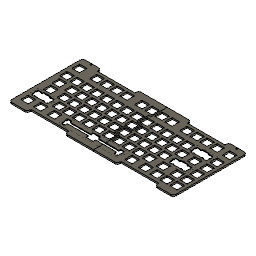
Plate (Autodesk Fusion 360 design; units mm, degrees)
part number: 2026-05-10-17-46-24-524
Autodesk Fusion 360 part; units mm, degrees
(part 1 of 4)
sketch "Plate May 11 2026" plane through (0, 0, 0) normal (0, 0, 1) x (1, 0, 0)
  line L0 (3.025, -2.525) -> (16.025, -2.525)
  line L1 (3.025, -16.525) -> (16.025, -16.525)
  line L2 (2.525, -3.025) -> (2.525, -16.025)
  line L3 (16.525, -3.025) -> (16.525, -16.025)
  arc A0 (3.025, -2.525) -> (2.525, -3.025) centre (3.025, -3.025) ccw
  arc A1 (16.525, -3.025) -> (16.025, -2.525) centre (16.025, -3.025) ccw
  arc A2 (2.525, -16.025) -> (3.025, -16.525) centre (3.025, -16.025) ccw
  arc A3 (16.025, -16.525) -> (16.525, -16.025) centre (16.025, -16.025) ccw
  line L4 (36.3625, -2.525) -> (49.3625, -2.525)
  line L5 (36.3625, -16.525) -> (49.3625, -16.525)
  line L6 (35.8625, -3.025) -> (35.8625, -16.025)
  line L7 (49.8625, -3.025) -> (49.8625, -16.025)
  arc A4 (36.3625, -2.525) -> (35.8625, -3.025) centre (36.3625, -3.025) ccw
  arc A5 (49.8625, -3.025) -> (49.3625, -2.525) centre (49.3625, -3.025) ccw
  arc A6 (35.8625, -16.025) -> (36.3625, -16.525) centre (36.3625, -16.025) ccw
  arc A7 (49.3625, -16.525) -> (49.8625, -16.025) centre (49.3625, -16.025) ccw
  line L8 (55.4125, -2.525) -> (68.4125, -2.525)
  line L9 (55.4125, -16.525) -> (68.4125, -16.525)
  line L10 (54.9125, -3.025) -> (54.9125, -16.025)
  line L11 (68.9125, -3.025) -> (68.9125, -16.025)
  arc A8 (55.4125, -2.525) -> (54.9125, -3.025) centre (55.4125, -3.025) ccw
  arc A9 (68.9125, -3.025) -> (68.4125, -2.525) centre (68.4125, -3.025) ccw
  arc A10 (54.9125, -16.025) -> (55.4125, -16.525) centre (55.4125, -16.025) ccw
  arc A11 (68.4125, -16.525) -> (68.9125, -16.025) centre (68.4125, -16.025) ccw
  line L12 (74.4625, -2.525) -> (87.4625, -2.525)
  line L13 (74.4625, -16.525) -> (87.4625, -16.525)
  line L14 (73.9625, -3.025) -> (73.9625, -16.025)
  line L15 (87.9625, -3.025) -> (87.9625, -16.025)
  arc A12 (74.4625, -2.525) -> (73.9625, -3.025) centre (74.4625, -3.025) ccw
  arc A13 (87.9625, -3.025) -> (87.4625, -2.525) centre (87.4625, -3.025) ccw
  arc A14 (73.9625, -16.025) -> (74.4625, -16.525) centre (74.4625, -16.025) ccw
  arc A15 (87.4625, -16.525) -> (87.9625, -16.025) centre (87.4625, -16.025) ccw
  line L16 (93.5125, -2.525) -> (106.5125, -2.525)
  line L17 (93.5125, -16.525) -> (106.5125, -16.525)
  line L18 (93.0125, -3.025) -> (93.0125, -16.025)
  line L19 (107.0125, -3.025) -> (107.0125, -16.025)
  arc A16 (93.5125, -2.525) -> (93.0125, -3.025) centre (93.5125, -3.025) ccw
  arc A17 (107.0125, -3.025) -> (106.5125, -2.525) centre (106.5125, -3.025) ccw
  arc A18 (93.0125, -16.025) -> (93.5125, -16.525) centre (93.5125, -16.025) ccw
  arc A19 (106.5125, -16.525) -> (107.0125, -16.025) centre (106.5125, -16.025) ccw
  line L20 (122.0875, -2.525) -> (135.0875, -2.525)
  line L21 (122.0875, -16.525) -> (135.0875, -16.525)
  line L22 (121.5875, -3.025) -> (121.5875, -16.025)
  line L23 (135.5875, -3.025) -> (135.5875, -16.025)
  arc A20 (122.0875, -2.525) -> (121.5875, -3.025) centre (122.0875, -3.025) ccw
  arc A21 (135.5875, -3.025) -> (135.0875, -2.525) centre (135.0875, -3.025) ccw
  arc A22 (121.5875, -16.025) -> (122.0875, -16.525) centre (122.0875, -16.025) ccw
  arc A23 (135.0875, -16.525) -> (135.5875, -16.025) centre (135.0875, -16.025) ccw
  line L24 (141.1375, -2.525) -> (154.1375, -2.525)
  line L25 (141.1375, -16.525) -> (154.1375, -16.525)
  line L26 (140.6375, -3.025) -> (140.6375, -16.025)
  line L27 (154.6375, -3.025) -> (154.6375, -16.025)
  arc A24 (141.1375, -2.525) -> (140.6375, -3.025) centre (141.1375, -3.025) ccw
  arc A25 (154.6375, -3.025) -> (154.1375, -2.525) centre (154.1375, -3.025) ccw
  arc A26 (140.6375, -16.025) -> (141.1375, -16.525) centre (141.1375, -16.025) ccw
  arc A27 (154.1375, -16.525) -> (154.6375, -16.025) centre (154.1375, -16.025) ccw
  line L28 (160.1875, -2.525) -> (173.1875, -2.525)
  line L29 (160.1875, -16.525) -> (173.1875, -16.525)
  line L30 (159.6875, -3.025) -> (159.6875, -16.025)
  line L31 (173.6875, -3.025) -> (173.6875, -16.025)
  arc A28 (160.1875, -2.525) -> (159.6875, -3.025) centre (160.1875, -3.025) ccw
  arc A29 (173.6875, -3.025) -> (173.1875, -2.525) centre (173.1875, -3.025) ccw
  arc A30 (159.6875, -16.025) -> (160.1875, -16.525) centre (160.1875, -16.025) ccw
  arc A31 (173.1875, -16.525) -> (173.6875, -16.025) centre (173.1875, -16.025) ccw
  line L32 (179.2375, -2.525) -> (192.2375, -2.525)
  line L33 (179.2375, -16.525) -> (192.2375, -16.525)
  line L34 (178.7375, -3.025) -> (178.7375, -16.025)
  line L35 (192.7375, -3.025) -> (192.7375, -16.025)
  arc A32 (179.2375, -2.525) -> (178.7375, -3.025) centre (179.2375, -3.025) ccw
  arc A33 (192.7375, -3.025) -> (192.2375, -2.525) centre (192.2375, -3.025) ccw
  arc A34 (178.7375, -16.025) -> (179.2375, -16.525) centre (179.2375, -16.025) ccw
  arc A35 (192.2375, -16.525) -> (192.7375, -16.025) centre (192.2375, -16.025) ccw
  line L36 (207.8125, -2.525) -> (220.8125, -2.525)
  line L37 (207.8125, -16.525) -> (220.8125, -16.525)
  line L38 (207.3125, -3.025) -> (207.3125, -16.025)
  line L39 (221.3125, -3.025) -> (221.3125, -16.025)
  arc A36 (207.8125, -2.525) -> (207.3125, -3.025) centre (207.8125, -3.025) ccw
  arc A37 (221.3125, -3.025) -> (220.8125, -2.525) centre (220.8125, -3.025) ccw
  arc A38 (207.3125, -16.025) -> (207.8125, -16.525) centre (207.8125, -16.025) ccw
  arc A39 (220.8125, -16.525) -> (221.3125, -16.025) centre (220.8125, -16.025) ccw
  line L40 (226.8625, -2.525) -> (239.8625, -2.525)
  line L41 (226.8625, -16.525) -> (239.8625, -16.525)
  line L42 (226.3625, -3.025) -> (226.3625, -16.025)
  line L43 (240.3625, -3.025) -> (240.3625, -16.025)
  arc A40 (226.8625, -2.525) -> (226.3625, -3.025) centre (226.8625, -3.025) ccw
  arc A41 (240.3625, -3.025) -> (239.8625, -2.525) centre (239.8625, -3.025) ccw
  arc A42 (226.3625, -16.025) -> (226.8625, -16.525) centre (226.8625, -16.025) ccw
  arc A43 (239.8625, -16.525) -> (240.3625, -16.025) centre (239.8625, -16.025) ccw
  line L44 (245.9125, -2.525) -> (258.9125, -2.525)
  line L45 (245.9125, -16.525) -> (258.9125, -16.525)
  line L46 (245.4125, -3.025) -> (245.4125, -16.025)
  line L47 (259.4125, -3.025) -> (259.4125, -16.025)
  arc A44 (245.9125, -2.525) -> (245.4125, -3.025) centre (245.9125, -3.025) ccw
  arc A45 (259.4125, -3.025) -> (258.9125, -2.525) centre (258.9125, -3.025) ccw
  arc A46 (245.4125, -16.025) -> (245.9125, -16.525) centre (245.9125, -16.025) ccw
  arc A47 (258.9125, -16.525) -> (259.4125, -16.025) centre (258.9125, -16.025) ccw
  line L48 (264.9625, -2.525) -> (277.9625, -2.525)
  line L49 (264.9625, -16.525) -> (277.9625, -16.525)
  line L50 (264.4625, -3.025) -> (264.4625, -16.025)
  line L51 (278.4625, -3.025) -> (278.4625, -16.025)
  arc A48 (264.9625, -2.525) -> (264.4625, -3.025) centre (264.9625, -3.025) ccw
  arc A49 (278.4625, -3.025) -> (277.9625, -2.525) centre (277.9625, -3.025) ccw
  arc A50 (264.4625, -16.025) -> (264.9625, -16.525) centre (264.9625, -16.025) ccw
  arc A51 (277.9625, -16.525) -> (278.4625, -16.025) centre (277.9625, -16.025) ccw
  line L52 (288.775, -2.5211) -> (301.775, -2.521)
  line L53 (288.775, -16.5282) -> (301.775, -16.5283)
  line L54 (288.239, -3.025) -> (288.2473, -16.025)
  line L55 (302.2755, -3.025) -> (302.2758, -16.025)
  arc A52 (288.775, -2.5211) -> (288.239, -3.025) centre (288.7579, -3.04) ccw
  arc A53 (302.2755, -3.025) -> (301.775, -2.521) centre (301.7743, -3.0222) ccw
  arc A54 (288.2473, -16.025) -> (288.775, -16.5282) centre (288.7619, -16.0136) ccw
  arc A55 (301.775, -16.5283) -> (302.2758, -16.025) centre (301.7745, -16.0271) ccw
  line L56 (3.025, -26.3375) -> (16.025, -26.3375)
  line L57 (3.025, -40.3375) -> (16.025, -40.3375)
  line L58 (2.525, -26.8375) -> (2.525, -39.8375)
  line L59 (16.525, -26.8375) -> (16.525, -39.8375)
  arc A56 (3.025, -26.3375) -> (2.525, -26.8375) centre (3.025, -26.8375) ccw
  arc A57 (16.525, -26.8375) -> (16.025, -26.3375) centre (16.025, -26.8375) ccw
  arc A58 (2.525, -39.8375) -> (3.025, -40.3375) centre (3.025, -39.8375) ccw
  arc A59 (16.025, -40.3375) -> (16.525, -39.8375) centre (16.025, -39.8375) ccw
  line L60 (22.075, -26.3375) -> (35.075, -26.3375)
  line L61 (22.075, -40.3375) -> (35.075, -40.3375)
  line L62 (21.575, -26.8375) -> (21.575, -39.8375)
  line L63 (35.575, -26.8375) -> (35.575, -39.8375)
  arc A60 (22.075, -26.3375) -> (21.575, -26.8375) centre (22.075, -26.8375) ccw
  arc A61 (35.575, -26.8375) -> (35.075, -26.3375) centre (35.075, -26.8375) ccw
  arc A62 (21.575, -39.8375) -> (22.075, -40.3375) centre (22.075, -39.8375) ccw
  arc A63 (35.075, -40.3375) -> (35.575, -39.8375) centre (35.075, -39.8375) ccw
  line L64 (41.125, -26.3375) -> (54.125, -26.3375)
  line L65 (41.125, -40.3375) -> (54.125, -40.3375)
  line L66 (40.625, -26.8375) -> (40.625, -39.8375)
  line L67 (54.625, -26.8375) -> (54.625, -39.8375)
  arc A64 (41.125, -26.3375) -> (40.625, -26.8375) centre (41.125, -26.8375) ccw
  arc A65 (54.625, -26.8375) -> (54.125, -26.3375) centre (54.125, -26.8375) ccw
  arc A66 (40.625, -39.8375) -> (41.125, -40.3375) centre (41.125, -39.8375) ccw
  arc A67 (54.125, -40.3375) -> (54.625, -39.8375) centre (54.125, -39.8375) ccw
  line L68 (60.175, -26.3375) -> (73.175, -26.3375)
  line L69 (60.175, -40.3375) -> (73.175, -40.3375)
  line L70 (59.675, -26.8375) -> (59.675, -39.8375)
  line L71 (73.675, -26.8375) -> (73.675, -39.8375)
  arc A68 (60.175, -26.3375) -> (59.675, -26.8375) centre (60.175, -26.8375) ccw
  arc A69 (73.675, -26.8375) -> (73.175, -26.3375) centre (73.175, -26.8375) ccw
  arc A70 (59.675, -39.8375) -> (60.175, -40.3375) centre (60.175, -39.8375) ccw
  arc A71 (73.175, -40.3375) -> (73.675, -39.8375) centre (73.175, -39.8375) ccw
  line L72 (79.225, -26.3375) -> (92.225, -26.3375)
  line L73 (79.225, -40.3375) -> (92.225, -40.3375)
  line L74 (78.725, -26.8375) -> (78.725, -39.8375)
  line L75 (92.725, -26.8375) -> (92.725, -39.8375)
  arc A72 (79.225, -26.3375) -> (78.725, -26.8375) centre (79.225, -26.8375) ccw
  arc A73 (92.725, -26.8375) -> (92.225, -26.3375) centre (92.225, -26.8375) ccw
  arc A74 (78.725, -39.8375) -> (79.225, -40.3375) centre (79.225, -39.8375) ccw
  arc A75 (92.225, -40.3375) -> (92.725, -39.8375) centre (92.225, -39.8375) ccw
  line L76 (98.275, -26.3375) -> (111.275, -26.3375)
  line L77 (98.275, -40.3375) -> (111.275, -40.3375)
  line L78 (97.775, -26.8375) -> (97.775, -39.8375)
  line L79 (111.775, -26.8375) -> (111.775, -39.8375)
  arc A76 (98.275, -26.3375) -> (97.775, -26.8375) centre (98.275, -26.8375) ccw
  arc A77 (111.775, -26.8375) -> (111.275, -26.3375) centre (111.275, -26.8375) ccw
  arc A78 (97.775, -39.8375) -> (98.275, -40.3375) centre (98.275, -39.8375) ccw
  arc A79 (111.275, -40.3375) -> (111.775, -39.8375) centre (111.275, -39.8375) ccw
  line L80 (117.325, -26.3375) -> (130.325, -26.3375)
  line L81 (117.325, -40.3375) -> (130.325, -40.3375)
  line L82 (116.825, -26.8375) -> (116.825, -39.8375)
  line L83 (130.825, -26.8375) -> (130.825, -39.8375)
  arc A80 (117.325, -26.3375) -> (116.825, -26.8375) centre (117.325, -26.8375) ccw
  arc A81 (130.825, -26.8375) -> (130.325, -26.3375) centre (130.325, -26.8375) ccw
  arc A82 (116.825, -39.8375) -> (117.325, -40.3375) centre (117.325, -39.8375) ccw
  arc A83 (130.325, -40.3375) -> (130.825, -39.8375) centre (130.325, -39.8375) ccw
  line L84 (136.375, -26.3375) -> (149.375, -26.3375)
  line L85 (136.375, -40.3375) -> (149.375, -40.3375)
  line L86 (135.875, -26.8375) -> (135.875, -39.8375)
  line L87 (149.875, -26.8375) -> (149.875, -39.8375)
  arc A84 (136.375, -26.3375) -> (135.875, -26.8375) centre (136.375, -26.8375) ccw
  arc A85 (149.875, -26.8375) -> (149.375, -26.3375) centre (149.375, -26.8375) ccw
  arc A86 (135.875, -39.8375) -> (136.375, -40.3375) centre (136.375, -39.8375) ccw
  arc A87 (149.375, -40.3375) -> (149.875, -39.8375) centre (149.375, -39.8375) ccw
  line L88 (155.425, -26.3375) -> (168.425, -26.3375)
  line L89 (155.425, -40.3375) -> (168.425, -40.3375)
  line L90 (154.925, -26.8375) -> (154.925, -39.8375)
  line L91 (168.925, -26.8375) -> (168.925, -39.8375)
  arc A88 (155.425, -26.3375) -> (154.925, -26.8375) centre (155.425, -26.8375) ccw
  arc A89 (168.925, -26.8375) -> (168.425, -26.3375) centre (168.425, -26.8375) ccw
  arc A90 (154.925, -39.8375) -> (155.425, -40.3375) centre (155.425, -39.8375) ccw
  arc A91 (168.425, -40.3375) -> (168.925, -39.8375) centre (168.425, -39.8375) ccw
  line L92 (174.475, -26.3375) -> (187.475, -26.3375)
  line L93 (174.475, -40.3375) -> (187.475, -40.3375)
  line L94 (173.975, -26.8375) -> (173.975, -39.8375)
  line L95 (187.975, -26.8375) -> (187.975, -39.8375)
  arc A92 (174.475, -26.3375) -> (173.975, -26.8375) centre (174.475, -26.8375) ccw
  arc A93 (187.975, -26.8375) -> (187.475, -26.3375) centre (187.475, -26.8375) ccw
  arc A94 (173.975, -39.8375) -> (174.475, -40.3375) centre (174.475, -39.8375) ccw
  arc A95 (187.475, -40.3375) -> (187.975, -39.8375) centre (187.475, -39.8375) ccw
  line L96 (193.525, -26.3375) -> (206.525, -26.3375)
  line L97 (193.525, -40.3375) -> (206.525, -40.3375)
  line L98 (193.025, -26.8375) -> (193.025, -39.8375)
  line L99 (207.025, -26.8375) -> (207.025, -39.8375)
  arc A96 (193.525, -26.3375) -> (193.025, -26.8375) centre (193.525, -26.8375) ccw
  arc A97 (207.025, -26.8375) -> (206.525, -26.3375) centre (206.525, -26.8375) ccw
  arc A98 (193.025, -39.8375) -> (193.525, -40.3375) centre (193.525, -39.8375) ccw
  arc A99 (206.525, -40.3375) -> (207.025, -39.8375) centre (206.525, -39.8375) ccw
  line L100 (212.575, -26.3375) -> (225.575, -26.3375)
  line L101 (212.575, -40.3375) -> (225.575, -40.3375)
  line L102 (212.075, -26.8375) -> (212.075, -39.8375)
  line L103 (226.075, -26.8375) -> (226.075, -39.8375)
  arc A100 (212.575, -26.3375) -> (212.075, -26.8375) centre (212.575, -26.8375) ccw
  arc A101 (226.075, -26.8375) -> (225.575, -26.3375) centre (225.575, -26.8375) ccw
  arc A102 (212.075, -39.8375) -> (212.575, -40.3375) centre (212.575, -39.8375) ccw
  arc A103 (225.575, -40.3375) -> (226.075, -39.8375) centre (225.575, -39.8375) ccw
  line L104 (231.625, -26.3375) -> (244.625, -26.3375)
  line L105 (231.625, -40.3375) -> (244.625, -40.3375)
  line L106 (231.125, -26.8375) -> (231.125, -39.8375)
  line L107 (245.125, -26.8375) -> (245.125, -39.8375)
  arc A104 (231.625, -26.3375) -> (231.125, -26.8375) centre (231.625, -26.8375) ccw
  arc A105 (245.125, -26.8375) -> (244.625, -26.3375) centre (244.625, -26.8375) ccw
  arc A106 (231.125, -39.8375) -> (231.625, -40.3375) centre (231.625, -39.8375) ccw
  arc A107 (244.625, -40.3375) -> (245.125, -39.8375) centre (244.625, -39.8375) ccw
  line L108 (260.2, -26.3375) -> (273.2, -26.3375)
  line L109 (260.2, -40.3375) -> (273.2, -40.3375)
  line L110 (259.7, -26.8375) -> (259.7, -39.8375)
  line L111 (273.7, -26.8375) -> (273.7, -39.8375)
  arc A108 (260.2, -26.3375) -> (259.7, -26.8375) centre (260.2, -26.8375) ccw
  arc A109 (273.7, -26.8375) -> (273.2, -26.3375) centre (273.2, -26.8375) ccw
  arc A110 (259.7, -39.8375) -> (260.2, -40.3375) centre (260.2, -39.8375) ccw
  arc A111 (273.2, -40.3375) -> (273.7, -39.8375) centre (273.2, -39.8375) ccw
  line L112 (251.9346, -27.6479) -> (257.5894, -27.6479)
  line L113 (258.0894, -28.1479) -> (258.0894, -28.4607)
  line L114 (258.0894, -28.4607) -> (266.7, -28.4607)
  line L115 (266.7, -39.1541) -> (258.5894, -39.1541)
  line L116 (258.0894, -39.6541) -> (258.0894, -39.9415)
  line L117 (258.0894, -39.9415) -> (256.786, -39.9415)
  line L118 (256.286, -40.4415) -> (256.286, -40.6099)
  line L119 (255.786, -41.1099) -> (253.738, -41.1099)
  line L120 (253.238, -40.6099) -> (253.238, -40.4415)
  line L121 (252.738, -39.9415) -> (251.9346, -39.9415)
  line L122 (251.4346, -39.4415) -> (251.4346, -34.3455)
  line L123 (250.9346, -33.8455) -> (250.571, -33.8455)
  line L124 (250.571, -33.8455) -> (250.571, -31.5515)
  line L125 (251.071, -31.0515) -> (251.4346, -31.0515)
  line L126 (251.4346, -31.0515) -> (251.4346, -28.1479)
  arc A112 (258.0894, -28.1479) -> (257.5894, -27.6479) centre (257.5894, -28.1479) ccw
  arc A113 (258.5894, -39.1541) -> (258.0894, -39.6541) centre (258.5894, -39.6541) ccw
  arc A114 (256.786, -39.9415) -> (256.286, -40.4415) centre (256.786, -40.4415) ccw
  arc A115 (255.786, -41.1099) -> (256.286, -40.6099) centre (255.786, -40.6099) ccw
  arc A116 (253.238, -40.6099) -> (253.738, -41.1099) centre (253.738, -40.6099) ccw
  arc A117 (253.238, -40.4415) -> (252.738, -39.9415) centre (252.738, -40.4415) ccw
  arc A118 (251.4346, -39.4415) -> (251.9346, -39.9415) centre (251.9346, -39.4415) ccw
  arc A119 (251.4346, -34.3455) -> (250.9346, -33.8455) centre (250.9346, -34.3455) ccw
  arc A120 (251.071, -31.0515) -> (250.571, -31.5515) centre (251.071, -31.5515) ccw
  arc A121 (251.9346, -27.6479) -> (251.4346, -28.1479) centre (251.9346, -28.1479) ccw
  line L127 (281.4654, -27.6479) -> (275.8106, -27.6479)
  line L128 (275.3106, -28.1479) -> (275.3106, -28.4607)
  line L129 (275.3106, -28.4607) -> (266.7, -28.4607)
  line L130 (266.7, -39.1541) -> (274.8106, -39.1541)
  line L131 (275.3106, -39.6541) -> (275.3106, -39.9415)
  line L132 (275.3106, -39.9415) -> (276.614, -39.9415)
  line L133 (277.114, -40.4415) -> (277.114, -40.6099)
  line L134 (277.614, -41.1099) -> (279.662, -41.1099)
  line L135 (280.162, -40.6099) -> (280.162, -40.4415)
  line L136 (280.662, -39.9415) -> (281.4654, -39.9415)
  line L137 (281.9654, -39.4415) -> (281.9654, -34.3455)
  line L138 (282.4654, -33.8455) -> (282.829, -33.8455)
  line L139 (282.829, -33.8455) -> (282.829, -31.5515)
  line L140 (282.329, -31.0515) -> (281.9654, -31.0515)
  line L141 (281.9654, -31.0515) -> (281.9654, -28.1479)
  arc A122 (275.8106, -27.6479) -> (275.3106, -28.1479) centre (275.8106, -28.1479) ccw
  arc A123 (275.3106, -39.6541) -> (274.8106, -39.1541) centre (274.8106, -39.6541) ccw
  arc A124 (277.114, -40.4415) -> (276.614, -39.9415) centre (276.614, -40.4415) ccw
  arc A125 (277.114, -40.6099) -> (277.614, -41.1099) centre (277.614, -40.6099) ccw
  arc A126 (279.662, -41.1099) -> (280.162, -40.6099) centre (279.662, -40.6099) ccw
  arc A127 (280.662, -39.9415) -> (280.162, -40.4415) centre (280.662, -40.4415) ccw
  arc A128 (281.4654, -39.9415) -> (281.9654, -39.4415) centre (281.4654, -39.4415) ccw
  arc A129 (282.4654, -33.8455) -> (281.9654, -34.3455) centre (282.4654, -34.3455) ccw
  arc A130 (282.829, -31.5515) -> (282.329, -31.0515) centre (282.329, -31.5515) ccw
  arc A131 (281.9654, -28.1479) -> (281.4654, -27.6479) centre (281.4654, -28.1479) ccw
  line L142 (288.775, -26.3375) -> (301.775, -26.3375)
  line L143 (288.775, -40.3375) -> (301.775, -40.3375)
  line L144 (288.275, -26.8375) -> (288.275, -39.8375)
  line L145 (302.275, -26.8375) -> (302.275, -39.8375)
  arc A132 (288.775, -26.3375) -> (288.275, -26.8375) centre (288.775, -26.8375) ccw
  arc A133 (302.275, -26.8375) -> (301.775, -26.3375) centre (301.775, -26.8375) ccw
  arc A134 (288.275, -39.8375) -> (288.775, -40.3375) centre (288.775, -39.8375) ccw
  arc A135 (301.775, -40.3375) -> (302.275, -39.8375) centre (301.775, -39.8375) ccw
  line L146 (7.7875, -45.3875) -> (20.7875, -45.3875)
  line L147 (7.7875, -59.3875) -> (20.7875, -59.3875)
  line L148 (7.2875, -45.8875) -> (7.2875, -58.8875)
  line L149 (21.2875, -45.8875) -> (21.2875, -58.8875)
  arc A136 (7.7875, -45.3875) -> (7.2875, -45.8875) centre (7.7875, -45.8875) ccw
  arc A137 (21.2875, -45.8875) -> (20.7875, -45.3875) centre (20.7875, -45.8875) ccw
  arc A138 (7.2875, -58.8875) -> (7.7875, -59.3875) centre (7.7875, -58.8875) ccw
  arc A139 (20.7875, -59.3875) -> (21.2875, -58.8875) centre (20.7875, -58.8875) ccw
  line L150 (31.6, -45.3875) -> (44.6, -45.3875)
  line L151 (31.6, -59.3875) -> (44.6, -59.3875)
  line L152 (31.1, -45.8875) -> (31.1, -58.8875)
  line L153 (45.1, -45.8875) -> (45.1, -58.8875)
  arc A140 (31.6, -45.3875) -> (31.1, -45.8875) centre (31.6, -45.8875) ccw
  arc A141 (45.1, -45.8875) -> (44.6, -45.3875) centre (44.6, -45.8875) ccw
  arc A142 (31.1, -58.8875) -> (31.6, -59.3875) centre (31.6, -58.8875) ccw
  arc A143 (44.6, -59.3875) -> (45.1, -58.8875) centre (44.6, -58.8875) ccw
  line L154 (50.65, -45.3875) -> (63.65, -45.3875)
  line L155 (50.65, -59.3875) -> (63.65, -59.3875)
  line L156 (50.15, -45.8875) -> (50.15, -58.8875)
  line L157 (64.15, -45.8875) -> (64.15, -58.8875)
  arc A144 (50.65, -45.3875) -> (50.15, -45.8875) centre (50.65, -45.8875) ccw
  arc A145 (64.15, -45.8875) -> (63.65, -45.3875) centre (63.65, -45.8875) ccw
  arc A146 (50.15, -58.8875) -> (50.65, -59.3875) centre (50.65, -58.8875) ccw
  arc A147 (63.65, -59.3875) -> (64.15, -58.8875) centre (63.65, -58.8875) ccw
  line L158 (69.7, -45.3875) -> (82.7, -45.3875)
  line L159 (69.7, -59.3875) -> (82.7, -59.3875)
  line L160 (69.2, -45.8875) -> (69.2, -58.8875)
  line L161 (83.2, -45.8875) -> (83.2, -58.8875)
  arc A148 (69.7, -45.3875) -> (69.2, -45.8875) centre (69.7, -45.8875) ccw
  arc A149 (83.2, -45.8875) -> (82.7, -45.3875) centre (82.7, -45.8875) ccw
  arc A150 (69.2, -58.8875) -> (69.7, -59.3875) centre (69.7, -58.8875) ccw
  arc A151 (82.7, -59.3875) -> (83.2, -58.8875) centre (82.7, -58.8875) ccw
  line L162 (88.75, -45.3875) -> (101.75, -45.3875)
  line L163 (88.75, -59.3875) -> (101.75, -59.3875)
  line L164 (88.25, -45.8875) -> (88.25, -58.8875)
  line L165 (102.25, -45.8875) -> (102.25, -58.8875)
  arc A152 (88.75, -45.3875) -> (88.25, -45.8875) centre (88.75, -45.8875) ccw
  arc A153 (102.25, -45.8875) -> (101.75, -45.3875) centre (101.75, -45.8875) ccw
  arc A154 (88.25, -58.8875) -> (88.75, -59.3875) centre (88.75, -58.8875) ccw
  arc A155 (101.75, -59.3875) -> (102.25, -58.8875) centre (101.75, -58.8875) ccw
  line L166 (107.8, -45.3875) -> (120.8, -45.3875)
  line L167 (107.8, -59.3875) -> (120.8, -59.3875)
  line L168 (107.3, -45.8875) -> (107.3, -58.8875)
  line L169 (121.3, -45.8875) -> (121.3, -58.8875)
  arc A156 (107.8, -45.3875) -> (107.3, -45.8875) centre (107.8, -45.8875) ccw
  arc A157 (121.3, -45.8875) -> (120.8, -45.3875) centre (120.8, -45.8875) ccw
  arc A158 (107.3, -58.8875) -> (107.8, -59.3875) centre (107.8, -58.8875) ccw
  arc A159 (120.8, -59.3875) -> (121.3, -58.8875) centre (120.8, -58.8875) ccw
  line L170 (126.85, -45.3875) -> (139.85, -45.3875)
  line L171 (126.85, -59.3875) -> (139.85, -59.3875)
  line L172 (126.35, -45.8875) -> (126.35, -58.8875)
  line L173 (140.35, -45.8875) -> (140.35, -58.8875)
  arc A160 (126.85, -45.3875) -> (126.35, -45.8875) centre (126.85, -45.8875) ccw
  arc A161 (140.35, -45.8875) -> (139.85, -45.3875) centre (139.85, -45.8875) ccw
  arc A162 (126.35, -58.8875) -> (126.85, -59.3875) centre (126.85, -58.8875) ccw
  arc A163 (139.85, -59.3875) -> (140.35, -58.8875) centre (139.85, -58.8875) ccw
  line L174 (145.9, -45.3875) -> (158.9, -45.3875)
  line L175 (145.9, -59.3875) -> (158.9, -59.3875)
  line L176 (145.4, -45.8875) -> (145.4, -58.8875)
  line L177 (159.4, -45.8875) -> (159.4, -58.8875)
  arc A164 (145.9, -45.3875) -> (145.4, -45.8875) centre (145.9, -45.8875) ccw
  arc A165 (159.4, -45.8875) -> (158.9, -45.3875) centre (158.9, -45.8875) ccw
  arc A166 (145.4, -58.8875) -> (145.9, -59.3875) centre (145.9, -58.8875) ccw
  arc A167 (158.9, -59.3875) -> (159.4, -58.8875) centre (158.9, -58.8875) ccw
  line L178 (164.95, -45.3875) -> (177.95, -45.3875)
  line L179 (164.95, -59.3875) -> (177.95, -59.3875)
  line L180 (164.45, -45.8875) -> (164.45, -58.8875)
  line L181 (178.45, -45.8875) -> (178.45, -58.8875)
  arc A168 (164.95, -45.3875) -> (164.45, -45.8875) centre (164.95, -45.8875) ccw
  arc A169 (178.45, -45.8875) -> (177.95, -45.3875) centre (177.95, -45.8875) ccw
  arc A170 (164.45, -58.8875) -> (164.95, -59.3875) centre (164.95, -58.8875) ccw
  arc A171 (177.95, -59.3875) -> (178.45, -58.8875) centre (177.95, -58.8875) ccw
  line L182 (184, -45.3875) -> (197, -45.3875)
  line L183 (184, -59.3875) -> (197, -59.3875)
  line L184 (183.5, -45.8875) -> (183.5, -58.8875)
  line L185 (197.5, -45.8875) -> (197.5, -58.8875)
  arc A172 (184, -45.3875) -> (183.5, -45.8875) centre (184, -45.8875) ccw
  arc A173 (197.5, -45.8875) -> (197, -45.3875) centre (197, -45.8875) ccw
  arc A174 (183.5, -58.8875) -> (184, -59.3875) centre (184, -58.8875) ccw
  arc A175 (197, -59.3875) -> (197.5, -58.8875) centre (197, -58.8875) ccw
  line L186 (203.05, -45.3875) -> (216.05, -45.3875)
  line L187 (203.05, -59.3875) -> (216.05, -59.3875)
  line L188 (202.55, -45.8875) -> (202.55, -58.8875)
  line L189 (216.55, -45.8875) -> (216.55, -58.8875)
  arc A176 (203.05, -45.3875) -> (202.55, -45.8875) centre (203.05, -45.8875) ccw
  arc A177 (216.55, -45.8875) -> (216.05, -45.3875) centre (216.05, -45.8875) ccw
  arc A178 (202.55, -58.8875) -> (203.05, -59.3875) centre (203.05, -58.8875) ccw
  arc A179 (216.05, -59.3875) -> (216.55, -58.8875) centre (216.05, -58.8875) ccw
  line L190 (222.1, -45.3875) -> (235.1, -45.3875)
  line L191 (222.1, -59.3875) -> (235.1, -59.3875)
  line L192 (221.6, -45.8875) -> (221.6, -58.8875)
  line L193 (235.6, -45.8875) -> (235.6, -58.8875)
  arc A180 (222.1, -45.3875) -> (221.6, -45.8875) centre (222.1, -45.8875) ccw
  arc A181 (235.6, -45.8875) -> (235.1, -45.3875) centre (235.1, -45.8875) ccw
  arc A182 (221.6, -58.8875) -> (222.1, -59.3875) centre (222.1, -58.8875) ccw
  arc A183 (235.1, -59.3875) -> (235.6, -58.8875) centre (235.1, -58.8875) ccw
  line L194 (241.15, -45.3875) -> (254.15, -45.3875)
  line L195 (241.15, -59.3875) -> (254.15, -59.3875)
  line L196 (240.65, -45.8875) -> (240.65, -58.8875)
  line L197 (254.65, -45.8875) -> (254.65, -58.8875)
  arc A184 (241.15, -45.3875) -> (240.65, -45.8875) centre (241.15, -45.8875) ccw
  arc A185 (254.65, -45.8875) -> (254.15, -45.3875) centre (254.15, -45.8875) ccw
  arc A186 (240.65, -58.8875) -> (241.15, -59.3875) centre (241.15, -58.8875) ccw
  arc A187 (254.15, -59.3875) -> (254.65, -58.8875) centre (254.15, -58.8875) ccw
  line L198 (264.9625, -45.3875) -> (277.9625, -45.3875)
  line L199 (264.9625, -59.3875) -> (277.9625, -59.3875)
  line L200 (264.4625, -45.8875) -> (264.4625, -58.8875)
  line L201 (278.4625, -45.8875) -> (278.4625, -58.8875)
  arc A188 (264.9625, -45.3875) -> (264.4625, -45.8875) centre (264.9625, -45.8875) ccw
  arc A189 (278.4625, -45.8875) -> (277.9625, -45.3875) centre (277.9625, -45.8875) ccw
  arc A190 (264.4625, -58.8875) -> (264.9625, -59.3875) centre (264.9625, -58.8875) ccw
  arc A191 (277.9625, -59.3875) -> (278.4625, -58.8875) centre (277.9625, -58.8875) ccw
  line L202 (288.775, -45.3875) -> (301.775, -45.3875)
  line L203 (288.775, -59.3875) -> (301.775, -59.3875)
  line L204 (288.275, -45.8875) -> (288.275, -58.8875)
  line L205 (302.275, -45.8875) -> (302.275, -58.8875)
  arc A192 (288.775, -45.3875) -> (288.275, -45.8875) centre (288.775, -45.8875) ccw
  arc A193 (302.275, -45.8875) -> (301.775, -45.3875) centre (301.775, -45.8875) ccw
  arc A194 (288.275, -58.8875) -> (288.775, -59.3875) centre (288.775, -58.8875) ccw
  arc A195 (301.775, -59.3875) -> (302.275, -58.8875) centre (301.775, -58.8875) ccw
  line L206 (10.1687, -64.4375) -> (23.1687, -64.4375)
  line L207 (10.1687, -78.4375) -> (23.1687, -78.4375)
  line L208 (9.6687, -64.9375) -> (9.6687, -77.9375)
  line L209 (23.6687, -64.9375) -> (23.6687, -77.9375)
  arc A196 (10.1687, -64.4375) -> (9.6688, -64.9375) centre (10.1687, -64.9375) ccw
  arc A197 (23.6687, -64.9375) -> (23.1687, -64.4375) centre (23.1687, -64.9375) ccw
  arc A198 (9.6687, -77.9375) -> (10.1687, -78.4375) centre (10.1687, -77.9375) ccw
  arc A199 (23.1687, -78.4375) -> (23.6687, -77.9375) centre (23.1687, -77.9375) ccw
  line L210 (36.3625, -64.4375) -> (49.3625, -64.4375)
  line L211 (36.3625, -78.4375) -> (49.3625, -78.4375)
  line L212 (35.8625, -64.9375) -> (35.8625, -77.9375)
  line L213 (49.8625, -64.9375) -> (49.8625, -77.9375)
  arc A200 (36.3625, -64.4375) -> (35.8625, -64.9375) centre (36.3625, -64.9375) ccw
  arc A201 (49.8625, -64.9375) -> (49.3625, -64.4375) centre (49.3625, -64.9375) ccw
  arc A202 (35.8625, -77.9375) -> (36.3625, -78.4375) centre (36.3625, -77.9375) ccw
  arc A203 (49.3625, -78.4375) -> (49.8625, -77.9375) centre (49.3625, -77.9375) ccw
  line L214 (55.4125, -64.4375) -> (68.4125, -64.4375)
  line L215 (55.4125, -78.4375) -> (68.4125, -78.4375)
  line L216 (54.9125, -64.9375) -> (54.9125, -77.9375)
  line L217 (68.9125, -64.9375) -> (68.9125, -77.9375)
  arc A204 (55.4125, -64.4375) -> (54.9125, -64.9375) centre (55.4125, -64.9375) ccw
  arc A205 (68.9125, -64.9375) -> (68.4125, -64.4375) centre (68.4125, -64.9375) ccw
  arc A206 (54.9125, -77.9375) -> (55.4125, -78.4375) centre (55.4125, -77.9375) ccw
  arc A207 (68.4125, -78.4375) -> (68.9125, -77.9375) centre (68.4125, -77.9375) ccw
  line L218 (74.4625, -64.4375) -> (87.4625, -64.4375)
  line L219 (74.4625, -78.4375) -> (87.4625, -78.4375)
  line L220 (73.9625, -64.9375) -> (73.9625, -77.9375)
  line L221 (87.9625, -64.9375) -> (87.9625, -77.9375)
  arc A208 (74.4625, -64.4375) -> (73.9625, -64.9375) centre (74.4625, -64.9375) ccw
  arc A209 (87.9625, -64.9375) -> (87.4625, -64.4375) centre (87.4625, -64.9375) ccw
  arc A210 (73.9625, -77.9375) -> (74.4625, -78.4375) centre (74.4625, -77.9375) ccw
  arc A211 (87.4625, -78.4375) -> (87.9625, -77.9375) centre (87.4625, -77.9375) ccw
  line L222 (93.5125, -64.4375) -> (106.5125, -64.4375)
  line L223 (93.5125, -78.4375) -> (106.5125, -78.4375)
  line L224 (93.0125, -64.9375) -> (93.0125, -77.9375)
  line L225 (107.0125, -64.9375) -> (107.0125, -77.9375)
  arc A212 (93.5125, -64.4375) -> (93.0125, -64.9375) centre (93.5125, -64.9375) ccw
  arc A213 (107.0125, -64.9375) -> (106.5125, -64.4375) centre (106.5125, -64.9375) ccw
  arc A214 (93.0125, -77.9375) -> (93.5125, -78.4375) centre (93.5125, -77.9375) ccw
  arc A215 (106.5125, -78.4375) -> (107.0125, -77.9375) centre (106.5125, -77.9375) ccw
  line L226 (112.5625, -64.4375) -> (125.5625, -64.4375)
  line L227 (112.5625, -78.4375) -> (125.5625, -78.4375)
  line L228 (112.0625, -64.9375) -> (112.0625, -77.9375)
  line L229 (126.0625, -64.9375) -> (126.0625, -77.9375)
  arc A216 (112.5625, -64.4375) -> (112.0625, -64.9375) centre (112.5625, -64.9375) ccw
  arc A217 (126.0625, -64.9375) -> (125.5625, -64.4375) centre (125.5625, -64.9375) ccw
  arc A218 (112.0625, -77.9375) -> (112.5625, -78.4375) centre (112.5625, -77.9375) ccw
  arc A219 (125.5625, -78.4375) -> (126.0625, -77.9375) centre (125.5625, -77.9375) ccw
  line L230 (131.6125, -64.4375) -> (144.6125, -64.4375)
  line L231 (131.6125, -78.4375) -> (144.6125, -78.4375)
  line L232 (131.1125, -64.9375) -> (131.1125, -77.9375)
  line L233 (145.1125, -64.9375) -> (145.1125, -77.9375)
  arc A220 (131.6125, -64.4375) -> (131.1125, -64.9375) centre (131.6125, -64.9375) ccw
  arc A221 (145.1125, -64.9375) -> (144.6125, -64.4375) centre (144.6125, -64.9375) ccw
  arc A222 (131.1125, -77.9375) -> (131.6125, -78.4375) centre (131.6125, -77.9375) ccw
  arc A223 (144.6125, -78.4375) -> (145.1125, -77.9375) centre (144.6125, -77.9375) ccw
  line L234 (150.6625, -64.4375) -> (163.6625, -64.4375)
  line L235 (150.6625, -78.4375) -> (163.6625, -78.4375)
  line L236 (150.1625, -64.9375) -> (150.1625, -77.9375)
  line L237 (164.1625, -64.9375) -> (164.1625, -77.9375)
  arc A224 (150.6625, -64.4375) -> (150.1625, -64.9375) centre (150.6625, -64.9375) ccw
  arc A225 (164.1625, -64.9375) -> (163.6625, -64.4375) centre (163.6625, -64.9375) ccw
  arc A226 (150.1625, -77.9375) -> (150.6625, -78.4375) centre (150.6625, -77.9375) ccw
  arc A227 (163.6625, -78.4375) -> (164.1625, -77.9375) centre (163.6625, -77.9375) ccw
  line L238 (169.7125, -64.4375) -> (182.7125, -64.4375)
  line L239 (169.7125, -78.4375) -> (182.7125, -78.4375)
  line L240 (169.2125, -64.9375) -> (169.2125, -77.9375)
  line L241 (183.2125, -64.9375) -> (183.2125, -77.9375)
  arc A228 (169.7125, -64.4375) -> (169.2125, -64.9375) centre (169.7125, -64.9375) ccw
  arc A229 (183.2125, -64.9375) -> (182.7125, -64.4375) centre (182.7125, -64.9375) ccw
  arc A230 (169.2125, -77.9375) -> (169.7125, -78.4375) centre (169.7125, -77.9375) ccw
  arc A231 (182.7125, -78.4375) -> (183.2125, -77.9375) centre (182.7125, -77.9375) ccw
  line L242 (188.7625, -64.4375) -> (201.7625, -64.4375)
  line L243 (188.7625, -78.4375) -> (201.7625, -78.4375)
  line L244 (188.2625, -64.9375) -> (188.2625, -77.9375)
  line L245 (202.2625, -64.9375) -> (202.2625, -77.9375)
  arc A232 (188.7625, -64.4375) -> (188.2625, -64.9375) centre (188.7625, -64.9375) ccw
  arc A233 (202.2625, -64.9375) -> (201.7625, -64.4375) centre (201.7625, -64.9375) ccw
  arc A234 (188.2625, -77.9375) -> (188.7625, -78.4375) centre (188.7625, -77.9375) ccw
  arc A235 (201.7625, -78.4375) -> (202.2625, -77.9375) centre (201.7625, -77.9375) ccw
  line L246 (207.8125, -64.4375) -> (220.8125, -64.4375)
  line L247 (207.8125, -78.4375) -> (220.8125, -78.4375)
  line L248 (207.3125, -64.9375) -> (207.3125, -77.9375)
  line L249 (221.3125, -64.9375) -> (221.3125, -77.9375)
  arc A236 (207.8125, -64.4375) -> (207.3125, -64.9375) centre (207.8125, -64.9375) ccw
  arc A237 (221.3125, -64.9375) -> (220.8125, -64.4375) centre (220.8125, -64.9375) ccw
  arc A238 (207.3125, -77.9375) -> (207.8125, -78.4375) centre (207.8125, -77.9375) ccw
  arc A239 (220.8125, -78.4375) -> (221.3125, -77.9375) centre (220.8125, -77.9375) ccw
  line L250 (226.8625, -64.4375) -> (239.8625, -64.4375)
  line L251 (226.8625, -78.4375) -> (239.8625, -78.4375)
  line L252 (226.3625, -64.9375) -> (226.3625, -77.9375)
  line L253 (240.3625, -64.9375) -> (240.3625, -77.9375)
  arc A240 (226.8625, -64.4375) -> (226.3625, -64.9375) centre (226.8625, -64.9375) ccw
  arc A241 (240.3625, -64.9375) -> (239.8625, -64.4375) centre (239.8625, -64.9375) ccw
  arc A242 (226.3625, -77.9375) -> (226.8625, -78.4375) centre (226.8625, -77.9375) ccw
  arc A243 (239.8625, -78.4375) -> (240.3625, -77.9375) centre (239.8625, -77.9375) ccw
  line L254 (257.8188, -64.4375) -> (270.8188, -64.4375)
  line L255 (257.8188, -78.4375) -> (270.8188, -78.4375)
  line L256 (257.3188, -64.9375) -> (257.3188, -77.9375)
  line L257 (271.3188, -64.9375) -> (271.3188, -77.9375)
  arc A244 (257.8188, -64.4375) -> (257.3188, -64.9375) centre (257.8188, -64.9375) ccw
  arc A245 (271.3188, -64.9375) -> (270.8188, -64.4375) centre (270.8188, -64.9375) ccw
  arc A246 (257.3188, -77.9375) -> (257.8188, -78.4375) centre (257.8188, -77.9375) ccw
  arc A247 (270.8188, -78.4375) -> (271.3188, -77.9375) centre (270.8188, -77.9375) ccw
  line L258 (249.5534, -65.7479) -> (255.2081, -65.7479)
  line L259 (255.7081, -66.2479) -> (255.7081, -66.5607)
  line L260 (255.7081, -66.5607) -> (264.3188, -66.5607)
  line L261 (264.3188, -77.2541) -> (256.2081, -77.2541)
  line L262 (255.7081, -77.7541) -> (255.7081, -78.0415)
  line L263 (255.7081, -78.0415) -> (254.4048, -78.0415)
  line L264 (253.9048, -78.5415) -> (253.9048, -78.7099)
  line L265 (253.4048, -79.2099) -> (251.3568, -79.2099)
  line L266 (250.8568, -78.7099) -> (250.8568, -78.5415)
  line L267 (250.3568, -78.0415) -> (249.5534, -78.0415)
  line L268 (249.0534, -77.5415) -> (249.0534, -72.4455)
  line L269 (248.5533, -71.9455) -> (248.1898, -71.9455)
  line L270 (248.1898, -71.9455) -> (248.1898, -69.6515)
  line L271 (248.6898, -69.1515) -> (249.0534, -69.1515)
  line L272 (249.0534, -69.1515) -> (249.0534, -66.2479)
  arc A248 (255.7081, -66.2479) -> (255.2081, -65.7479) centre (255.2081, -66.2479) ccw
  arc A249 (256.2081, -77.2541) -> (255.7081, -77.7541) centre (256.2081, -77.7541) ccw
  arc A250 (254.4048, -78.0415) -> (253.9048, -78.5415) centre (254.4048, -78.5415) ccw
  arc A251 (253.4048, -79.2099) -> (253.9048, -78.7099) centre (253.4048, -78.7099) ccw
  arc A252 (250.8568, -78.7099) -> (251.3568, -79.2099) centre (251.3568, -78.7099) ccw
  arc A253 (250.8568, -78.5415) -> (250.3568, -78.0415) centre (250.3568, -78.5415) ccw
  arc A254 (249.0534, -77.5415) -> (249.5534, -78.0415) centre (249.5534, -77.5415) ccw
  arc A255 (249.0533, -72.4455) -> (248.5533, -71.9455) centre (248.5533, -72.4455) ccw
  arc A256 (248.6898, -69.1515) -> (248.1898, -69.6515) centre (248.6898, -69.6515) ccw
  arc A257 (249.5534, -65.7479) -> (249.0534, -66.2479) centre (249.5534, -66.2479) ccw
  line L273 (279.0842, -65.7479) -> (273.4293, -65.7479)
  line L274 (272.9293, -66.2479) -> (272.9293, -66.5607)
  line L275 (272.9293, -66.5607) -> (264.3188, -66.5607)
  line L276 (264.3188, -77.2541) -> (272.4293, -77.2541)
  line L277 (272.9293, -77.7541) -> (272.9293, -78.0415)
  line L278 (272.9293, -78.0415) -> (274.2328, -78.0415)
  line L279 (274.7328, -78.5415) -> (274.7328, -78.7099)
  line L280 (275.2328, -79.2099) -> (277.2808, -79.2099)
  line L281 (277.7808, -78.7099) -> (277.7808, -78.5415)
  line L282 (278.2808, -78.0415) -> (279.0842, -78.0415)
  line L283 (279.5842, -77.5415) -> (279.5842, -72.4455)
  line L284 (280.0842, -71.9455) -> (280.4477, -71.9455)
  line L285 (280.4478, -71.9455) -> (280.4478, -69.6515)
  line L286 (279.9477, -69.1515) -> (279.5842, -69.1515)
  line L287 (279.5842, -69.1515) -> (279.5842, -66.2479)
  arc A258 (273.4293, -65.7479) -> (272.9293, -66.2479) centre (273.4293, -66.2479) ccw
  arc A259 (272.9293, -77.7541) -> (272.4293, -77.2541) centre (272.4293, -77.7541) ccw
  arc A260 (274.7328, -78.5415) -> (274.2328, -78.0415) centre (274.2328, -78.5415) ccw
  arc A261 (274.7328, -78.7099) -> (275.2328, -79.2099) centre (275.2328, -78.7099) ccw
  arc A262 (277.2808, -79.2099) -> (277.7808, -78.7099) centre (277.2808, -78.7099) ccw
  arc A263 (278.2808, -78.0415) -> (277.7808, -78.5415) centre (278.2808, -78.5415) ccw
  arc A264 (279.0842, -78.0415) -> (279.5842, -77.5415) centre (279.0842, -77.5415) ccw
  arc A265 (280.0842, -71.9455) -> (279.5842, -72.4455) centre (280.0842, -72.4455) ccw
  arc A266 (280.4477, -69.6515) -> (279.9477, -69.1515) centre (279.9477, -69.6515) ccw
  arc A267 (279.5842, -66.2479) -> (279.0842, -65.7479) centre (279.0842, -66.2479) ccw
  line L288 (288.775, -64.4375) -> (301.775, -64.4375)
  line L289 (288.775, -78.4375) -> (301.775, -78.4375)
  line L290 (288.275, -64.9375) -> (288.275, -77.9375)
  line L291 (302.275, -64.9375) -> (302.275, -77.9375)
  arc A268 (288.775, -64.4375) -> (288.275, -64.9375) centre (288.775, -64.9375) ccw
  arc A269 (302.275, -64.9375) -> (301.775, -64.4375) centre (301.775, -64.9375) ccw
  arc A270 (288.275, -77.9375) -> (288.775, -78.4375) centre (288.775, -77.9375) ccw
  arc A271 (301.775, -78.4375) -> (302.275, -77.9375) centre (301.775, -77.9375) ccw
  line L292 (14.9313, -83.4875) -> (27.9312, -83.4875)
  line L293 (14.9313, -97.4875) -> (27.9312, -97.4875)
  line L294 (14.4313, -83.9875) -> (14.4313, -96.9875)
  line L295 (28.4313, -83.9875) -> (28.4313, -96.9875)
  arc A272 (14.9313, -83.4875) -> (14.4313, -83.9875) centre (14.9313, -83.9875) ccw
  arc A273 (28.4313, -83.9875) -> (27.9312, -83.4875) centre (27.9312, -83.9875) ccw
  arc A274 (14.4313, -96.9875) -> (14.9313, -97.4875) centre (14.9313, -96.9875) ccw
  arc A275 (27.9312, -97.4875) -> (28.4313, -96.9875) centre (27.9312, -96.9875) ccw
  line L296 (6.6658, -84.7979) -> (12.3207, -84.7979)
  line L297 (12.8207, -85.2979) -> (12.8207, -85.6107)
  line L298 (12.8207, -85.6107) -> (21.4312, -85.6107)
  line L299 (21.4312, -96.3041) -> (13.3207, -96.3041)
  line L300 (12.8207, -96.8041) -> (12.8207, -97.0915)
  line L301 (12.8207, -97.0915) -> (11.5173, -97.0915)
  line L302 (11.0173, -97.5915) -> (11.0173, -97.7599)
  line L303 (10.5173, -98.2599) -> (8.4693, -98.2599)
  line L304 (7.9692, -97.7599) -> (7.9692, -97.5915)
  line L305 (7.4693, -97.0915) -> (6.6658, -97.0915)
  line L306 (6.1659, -96.5915) -> (6.1659, -91.4955)
  line L307 (5.6658, -90.9955) -> (5.3023, -90.9955)
  line L308 (5.3023, -90.9955) -> (5.3023, -88.7015)
  line L309 (5.8022, -88.2015) -> (6.1659, -88.2015)
  line L310 (6.1659, -88.2015) -> (6.1659, -85.2979)
  arc A276 (12.8207, -85.2979) -> (12.3207, -84.7979) centre (12.3207, -85.2979) ccw
  arc A277 (13.3207, -96.3041) -> (12.8206, -96.8041) centre (13.3207, -96.8041) ccw
  arc A278 (11.5173, -97.0915) -> (11.0173, -97.5915) centre (11.5173, -97.5915) ccw
  arc A279 (10.5173, -98.2599) -> (11.0173, -97.7599) centre (10.5173, -97.7599) ccw
  arc A280 (7.9693, -97.7599) -> (8.4693, -98.2599) centre (8.4693, -97.7599) ccw
  arc A281 (7.9692, -97.5915) -> (7.4693, -97.0915) centre (7.4693, -97.5915) ccw
  arc A282 (6.1659, -96.5915) -> (6.6658, -97.0915) centre (6.6658, -96.5915) ccw
  arc A283 (6.1659, -91.4955) -> (5.6658, -90.9955) centre (5.6658, -91.4955) ccw
  arc A284 (5.8022, -88.2015) -> (5.3022, -88.7015) centre (5.8022, -88.7015) ccw
  arc A285 (6.6658, -84.7979) -> (6.1658, -85.2979) centre (6.6658, -85.2979) ccw
  line L311 (36.1966, -84.7979) -> (30.5419, -84.7979)
  line L312 (30.0419, -85.2979) -> (30.0419, -85.6107)
  line L313 (30.0419, -85.6107) -> (21.4312, -85.6107)
  line L314 (21.4312, -96.3041) -> (29.5419, -96.3041)
  line L315 (30.0419, -96.8041) -> (30.0419, -97.0915)
  line L316 (30.0419, -97.0915) -> (31.3452, -97.0915)
  line L317 (31.8453, -97.5915) -> (31.8453, -97.7599)
  line L318 (32.3453, -98.2599) -> (34.3933, -98.2599)
  line L319 (34.8933, -97.7599) -> (34.8933, -97.5915)
  line L320 (35.3933, -97.0915) -> (36.1966, -97.0915)
  line L321 (36.6967, -96.5915) -> (36.6967, -91.4955)
  line L322 (37.1966, -90.9955) -> (37.5603, -90.9955)
  line L323 (37.5603, -90.9955) -> (37.5603, -88.7015)
  line L324 (37.0603, -88.2015) -> (36.6967, -88.2015)
  line L325 (36.6967, -88.2015) -> (36.6967, -85.2979)
  arc A286 (30.5419, -84.7979) -> (30.0418, -85.2979) centre (30.5419, -85.2979) ccw
  arc A287 (30.0419, -96.8041) -> (29.5419, -96.3041) centre (29.5419, -96.8041) ccw
  arc A288 (31.8453, -97.5915) -> (31.3452, -97.0915) centre (31.3452, -97.5915) ccw
  arc A289 (31.8453, -97.7599) -> (32.3453, -98.2599) centre (32.3453, -97.7599) ccw
  arc A290 (34.3933, -98.2599) -> (34.8933, -97.7599) centre (34.3933, -97.7599) ccw
  arc A291 (35.3933, -97.0915) -> (34.8933, -97.5915) centre (35.3933, -97.5915) ccw
  arc A292 (36.1966, -97.0915) -> (36.6967, -96.5915) centre (36.1966, -96.5915) ccw
  arc A293 (37.1966, -90.9955) -> (36.6966, -91.4955) centre (37.1966, -91.4955) ccw
  arc A294 (37.5603, -88.7015) -> (37.0603, -88.2015) centre (37.0603, -88.7015) ccw
  arc A295 (36.6966, -85.2979) -> (36.1966, -84.7979) centre (36.1966, -85.2979) ccw
  line L326 (45.8875, -83.4875) -> (58.8875, -83.4875)
  line L327 (45.8875, -97.4875) -> (58.8875, -97.4875)
  line L328 (45.3875, -83.9875) -> (45.3875, -96.9875)
  line L329 (59.3875, -83.9875) -> (59.3875, -96.9875)
  arc A296 (45.8875, -83.4875) -> (45.3875, -83.9875) centre (45.8875, -83.9875) ccw
  arc A297 (59.3875, -83.9875) -> (58.8875, -83.4875) centre (58.8875, -83.9875) ccw
  arc A298 (45.3875, -96.9875) -> (45.8875, -97.4875) centre (45.8875, -96.9875) ccw
  arc A299 (58.8875, -97.4875) -> (59.3875, -96.9875) centre (58.8875, -96.9875) ccw
  line L330 (64.9375, -83.4875) -> (77.9375, -83.4875)
  line L331 (64.9375, -97.4875) -> (77.9375, -97.4875)
  line L332 (64.4375, -83.9875) -> (64.4375, -96.9875)
  line L333 (78.4375, -83.9875) -> (78.4375, -96.9875)
  arc A300 (64.9375, -83.4875) -> (64.4375, -83.9875) centre (64.9375, -83.9875) ccw
  arc A301 (78.4375, -83.9875) -> (77.9375, -83.4875) centre (77.9375, -83.9875) ccw
  arc A302 (64.4375, -96.9875) -> (64.9375, -97.4875) centre (64.9375, -96.9875) ccw
  arc A303 (77.9375, -97.4875) -> (78.4375, -96.9875) centre (77.9375, -96.9875) ccw
  line L334 (83.9875, -83.4875) -> (96.9875, -83.4875)
  line L335 (83.9875, -97.4875) -> (96.9875, -97.4875)
  line L336 (83.4875, -83.9875) -> (83.4875, -96.9875)
  line L337 (97.4875, -83.9875) -> (97.4875, -96.9875)
  arc A304 (83.9875, -83.4875) -> (83.4875, -83.9875) centre (83.9875, -83.9875) ccw
  arc A305 (97.4875, -83.9875) -> (96.9875, -83.4875) centre (96.9875, -83.9875) ccw
  arc A306 (83.4875, -96.9875) -> (83.9875, -97.4875) centre (83.9875, -96.9875) ccw
  arc A307 (96.9875, -97.4875) -> (97.4875, -96.9875) centre (96.9875, -96.9875) ccw
  line L338 (103.0375, -83.4875) -> (116.0375, -83.4875)
  line L339 (103.0375, -97.4875) -> (116.0375, -97.4875)
  line L340 (102.5375, -83.9875) -> (102.5375, -96.9875)
  line L341 (116.5375, -83.9875) -> (116.5375, -96.9875)
  arc A308 (103.0375, -83.4875) -> (102.5375, -83.9875) centre (103.0375, -83.9875) ccw
  arc A309 (116.5375, -83.9875) -> (116.0375, -83.4875) centre (116.0375, -83.9875) ccw
  arc A310 (102.5375, -96.9875) -> (103.0375, -97.4875) centre (103.0375, -96.9875) ccw
  arc A311 (116.0375, -97.4875) -> (116.5375, -96.9875) centre (116.0375, -96.9875) ccw
  line L342 (122.0875, -83.4875) -> (135.0875, -83.4875)
  line L343 (122.0875, -97.4875) -> (135.0875, -97.4875)
  line L344 (121.5875, -83.9875) -> (121.5875, -96.9875)
  line L345 (135.5875, -83.9875) -> (135.5875, -96.9875)
  arc A312 (122.0875, -83.4875) -> (121.5875, -83.9875) centre (122.0875, -83.9875) ccw
  arc A313 (135.5875, -83.9875) -> (135.0875, -83.4875) centre (135.0875, -83.9875) ccw
  arc A314 (121.5875, -96.9875) -> (122.0875, -97.4875) centre (122.0875, -96.9875) ccw
  arc A315 (135.0875, -97.4875) -> (135.5875, -96.9875) centre (135.0875, -96.9875) ccw
  line L346 (141.1375, -83.4875) -> (154.1375, -83.4875)
  line L347 (141.1375, -97.4875) -> (154.1375, -97.4875)
  line L348 (140.6375, -83.9875) -> (140.6375, -96.9875)
  line L349 (154.6375, -83.9875) -> (154.6375, -96.9875)
  arc A316 (141.1375, -83.4875) -> (140.6375, -83.9875) centre (141.1375, -83.9875) ccw
  arc A317 (154.6375, -83.9875) -> (154.1375, -83.4875) centre (154.1375, -83.9875) ccw
  arc A318 (140.6375, -96.9875) -> (141.1375, -97.4875) centre (141.1375, -96.9875) ccw
  arc A319 (154.1375, -97.4875) -> (154.6375, -96.9875) centre (154.1375, -96.9875) ccw
  line L350 (160.1875, -83.4875) -> (173.1875, -83.4875)
  line L351 (160.1875, -97.4875) -> (173.1875, -97.4875)
  line L352 (159.6875, -83.9875) -> (159.6875, -96.9875)
  line L353 (173.6875, -83.9875) -> (173.6875, -96.9875)
  arc A320 (160.1875, -83.4875) -> (159.6875, -83.9875) centre (160.1875, -83.9875) ccw
  arc A321 (173.6875, -83.9875) -> (173.1875, -83.4875) centre (173.1875, -83.9875) ccw
  arc A322 (159.6875, -96.9875) -> (160.1875, -97.4875) centre (160.1875, -96.9875) ccw
  arc A323 (173.1875, -97.4875) -> (173.6875, -96.9875) centre (173.1875, -96.9875) ccw
  line L354 (179.2375, -83.4875) -> (192.2375, -83.4875)
  line L355 (179.2375, -97.4875) -> (192.2375, -97.4875)
  line L356 (178.7375, -83.9875) -> (178.7375, -96.9875)
  line L357 (192.7375, -83.9875) -> (192.7375, -96.9875)
  arc A324 (179.2375, -83.4875) -> (178.7375, -83.9875) centre (179.2375, -83.9875) ccw
  arc A325 (192.7375, -83.9875) -> (192.2375, -83.4875) centre (192.2375, -83.9875) ccw
  arc A326 (178.7375, -96.9875) -> (179.2375, -97.4875) centre (179.2375, -96.9875) ccw
  arc A327 (192.2375, -97.4875) -> (192.7375, -96.9875) centre (192.2375, -96.9875) ccw
  line L358 (198.2875, -83.4875) -> (211.2875, -83.4875)
  line L359 (198.2875, -97.4875) -> (211.2875, -97.4875)
  line L360 (197.7875, -83.9875) -> (197.7875, -96.9875)
  line L361 (211.7875, -83.9875) -> (211.7875, -96.9875)
  arc A328 (198.2875, -83.4875) -> (197.7875, -83.9875) centre (198.2875, -83.9875) ccw
  arc A329 (211.7875, -83.9875) -> (211.2875, -83.4875) centre (211.2875, -83.9875) ccw
  arc A330 (197.7875, -96.9875) -> (198.2875, -97.4875) centre (198.2875, -96.9875) ccw
  arc A331 (211.2875, -97.4875) -> (211.7875, -96.9875) centre (211.2875, -96.9875) ccw
  line L362 (217.3375, -83.4875) -> (230.3375, -83.4875)
  line L363 (217.3375, -97.4875) -> (230.3375, -97.4875)
  line L364 (216.8375, -83.9875) -> (216.8375, -96.9875)
  line L365 (230.8375, -83.9875) -> (230.8375, -96.9875)
  arc A332 (217.3375, -83.4875) -> (216.8375, -83.9875) centre (217.3375, -83.9875) ccw
  arc A333 (230.8375, -83.9875) -> (230.3375, -83.4875) centre (230.3375, -83.9875) ccw
  arc A334 (216.8375, -96.9875) -> (217.3375, -97.4875) centre (217.3375, -96.9875) ccw
  arc A335 (230.3375, -97.4875) -> (230.8375, -96.9875) centre (230.3375, -96.9875) ccw
  line L366 (243.5313, -83.4875) -> (256.5313, -83.4875)
  line L367 (243.5313, -97.4875) -> (256.5313, -97.4875)
  line L368 (243.0312, -83.9875) -> (243.0312, -96.9875)
  line L369 (257.0312, -83.9875) -> (257.0312, -96.9875)
  arc A336 (243.5313, -83.4875) -> (243.0313, -83.9875) centre (243.5313, -83.9875) ccw
  arc A337 (257.0312, -83.9875) -> (256.5312, -83.4875) centre (256.5312, -83.9875) ccw
  arc A338 (243.0313, -96.9875) -> (243.5313, -97.4875) centre (243.5313, -96.9875) ccw
  arc A339 (256.5312, -97.4875) -> (257.0312, -96.9875) centre (256.5312, -96.9875) ccw
  line L370 (269.725, -83.4875) -> (282.725, -83.4875)
  line L371 (269.725, -97.4875) -> (282.725, -97.4875)
  line L372 (269.225, -83.9875) -> (269.225, -96.9875)
  line L373 (283.225, -83.9875) -> (283.225, -96.9875)
  arc A340 (269.725, -83.4875) -> (269.225, -83.9875) centre (269.725, -83.9875) ccw
  arc A341 (283.225, -83.9875) -> (282.725, -83.4875) centre (282.725, -83.9875) ccw
  arc A342 (269.225, -96.9875) -> (269.725, -97.4875) centre (269.725, -96.9875) ccw
  arc A343 (282.725, -97.4875) -> (283.225, -96.9875) centre (282.725, -96.9875) ccw
  line L374 (288.775, -83.4875) -> (301.775, -83.4875)
  line L375 (288.775, -97.4875) -> (301.775, -97.4875)
  line L376 (288.275, -83.9875) -> (288.275, -96.9875)
  line L377 (302.275, -83.9875) -> (302.275, -96.9875)
  arc A344 (288.775, -83.4875) -> (288.275, -83.9875) centre (288.775, -83.9875) ccw
  arc A345 (302.275, -83.9875) -> (301.775, -83.4875) centre (301.775, -83.9875) ccw
  arc A346 (288.275, -96.9875) -> (288.775, -97.4875) centre (288.775, -96.9875) ccw